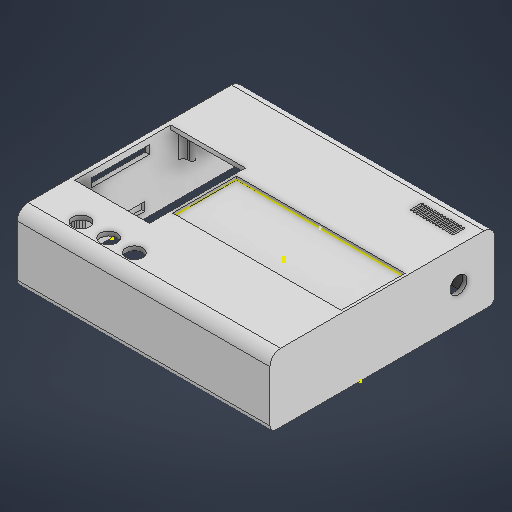
# Autodesk Inventor part: casereceptora
Saved by Autodesk Inventor 2026.1 (Build 301233020, 233B)
## iProperties
Created: 2025-11-04
Part Number: casereceptora
Material: Genérico
Document SubType Name: Modeling
Designer: luska
Density: 1 g/cm^3
Appearance: Padrão
Author: luska
## iProperties of the stored document casereceptora_3DPrint.ipt
Created: 2025-11-11
Part Number: casereceptora_3DPrint
Material: Genérico
Document SubType Name: Modeling
Designer: luska
Density: 1 g/cm^3
Appearance: Padrão
Author: luska
Autodesk Inventor part; units mm, degrees
ref_plane "YZ Plane" through (0, 0, 0) normal (1, 0, 0) x (0, 1, 0)
ref_plane "XZ Plane" through (0, 0, 0) normal (0, 1, 0) x (-1, 0, 0)
ref_plane "XY Plane" through (0, 0, 0) normal (0, 0, 1) x (1, 0, 0)
sketch "Esboço1" plane through (0, 0, 0) normal (0, 1, 0) x (-1, 0, 0)
  line L0 (82.792, 42.4072) -> (-35.708, 42.4072)
  line L1 (-35.708, 42.4072) -> (-35.708, -63.0628)
  line L2 (-35.708, -63.0628) -> (82.792, -63.0628)
  line L3 (82.792, -63.0628) -> (82.792, 42.4072)
  point P0 (0, 0)
  constraints: 8 end point, 2 parallel, 1 horizontal, 1 perpendicular
extrude "Extrusão1" add sketch "Esboço1" along normal blind 32
sketch "Esboço2" plane through (0, 0, 0) normal (0, -1, 0) x (1, 0, 0)
  line L0 (-80.792, 39.4072) -> (33.708, 39.4072)
  line L1 (33.708, 39.4072) -> (33.708, -60.0628)
  line L2 (33.708, -60.0628) -> (-80.792, -60.0628)
  line L3 (-80.792, -60.0628) -> (-80.792, 39.4072)
  line L4 (-82.792, -63.0628) -> (-82.792, 42.4072) projected
  line L5 (35.708, 42.4072) -> (35.708, -63.0628) projected
  line L6 (-82.792, 42.4072) -> (35.708, 42.4072) projected
  line L7 (35.708, -63.0628) -> (-82.792, -63.0628) projected
  point P0 (0, 0)
  constraints: 8 end point, 2 parallel, 1 horizontal, 1 perpendicular
extrude "Extrusão2" cut sketch "Esboço2" against normal blind 30 contours L0 L1 L2 L3
sketch "Esboço3" plane through (-82.792, 0, -63.0628) normal (-1, 0, 0) x (0, 0, 1)
  line L0 (24.47, 25) -> (14.47, 25)
  line L1 (14.47, 25) -> (14.47, 20)
  line L2 (14.47, 20) -> (24.47, 20)
  line L3 (24.47, 20) -> (24.47, 25)
  line L4 (0, 32) -> (105.47, 32) projected
  line L5 (0, 0) -> (0, 32) projected
  line L6 (45.47, 25) -> (72.47, 25)
  line L7 (72.47, 25) -> (72.47, 29)
  line L8 (72.47, 29) -> (45.47, 29)
  line L9 (45.47, 29) -> (45.47, 25)
  line L10 (105.47, 0) -> (105.47, 32) projected
  point P0 (63.0628, 0)
  point P1 (19.47, 25)
  point P2 (14.47, 22.5)
  point P3 (52.735, 32)
  point P4 (72.47, 27)
  point P5 (45.47, 27)
  dimension "d12" = 10
  dimension "d13" = 5
  dimension "d16" = 27
  dimension "d17" = 4
  dimension "d18" = 3
  dimension "d19" = 33
  dimension "d269" = 21
  dimension "d273" = 7
  constraints: 16 end point, 5 midpoint, 4 parallel, 2 horizontal, 2 perpendicular
  measures "d12" distance of L2.end L1.end
  measures "d13" distance of L1.end L0.end
  measures "d16" distance of L8.end L7.end
  measures "d17" distance of L7.end L6.end
  measures "d18" distance from line of point (52.735, 32) L8
  measures "d19" distance from line of L10 point (72.47, 27)
  measures "d269" distance from line of point (45.47, 27) L3
  measures "d273" distance between parallel lines of L4 L0
extrude "Extrusão3" cut sketch "Esboço3" against normal blind 2
sketch "Esboço4" plane through (0, 30, 0) normal (0, -1, 0) x (1, 0, 0)
  point P0 (0, 0)
sketch "Esboço5" plane through (0, 30, 0) normal (0, -1, 0) x (1, 0, 0)
  line L0 (-45.792, -27.5928) -> (-80.792, -27.5928)
  line L1 (-80.792, -27.5928) -> (-80.792, 17.4072)
  line L2 (-80.792, 17.4072) -> (-45.792, 17.4072)
  line L3 (-45.792, 17.4072) -> (-45.792, -27.5928)
  line L4 (-82.792, -63.0628) -> (-82.792, 42.4072) projected
  line L5 (-82.792, 42.4072) -> (35.708, 42.4072) projected
  line L6 (-80.792, 39.4072) -> (33.708, 39.4072) projected
  point P0 (0, 0)
  point P1 (-63.292, 17.4072)
  dimension "d22" = 35
  dimension "d23" = 45
  dimension "d24" = 2
  dimension "d268" = 22
  constraints: 8 end point, 2 parallel, 1 horizontal, 1 midpoint, 1 perpendicular
  measures "d22" distance of L1.end L2.end
  measures "d23" distance from line of point (-63.292, 17.407) L0
  measures "d24" distance between parallel lines of L4 L1
  measures "d268" distance between parallel lines of L6 L2
extrude "Extrusão4" cut sketch "Esboço5" against normal blind 2
sketch "Esboço6" plane through (0, 30, 0) normal (0, -1, 0) x (1, 0, 0)
  circle A0 centre (-78.392, 36.4072) radius 1.5
  line L0 (-80.792, -60.0628) -> (-80.792, 39.4072) projected
  line L1 (-80.792, 39.4072) -> (33.708, 39.4072) projected
  circle A1 centre (24.108, 35.4072) radius 1.25
  circle A2 centre (25.208, -54.0928) radius 1.25
  circle A3 centre (-77.792, -34.5928) radius 1.25
  line L2 (33.708, -60.0628) -> (-80.792, -60.0628) projected
  point P0 (0, 0)
  dimension "d28" = 3
  dimension "d29" = 2.4
  dimension "d30" = 3
  dimension "d32" = 2.5
  dimension "d33" = 2.5
  dimension "d34" = 2.5
  dimension "d35" = 4
  dimension "d39" = 3
  dimension "d249" = 102.5
  dimension "d250" = 71
  dimension "d251" = 89.5
  dimension "d261" = 106
  constraints: 4 centre point
  measures "d28" diameter of A0
  measures "d29" distance from line of L0 A0.centre
  measures "d30" distance from line of A0.centre L1
  measures "d32" diameter of A1
  measures "d33" diameter of A2
  measures "d34" diameter of A3
  measures "d35" distance from line of L1 A1.centre
  measures "d39" distance from line of L0 A3.centre
  measures "d249" horizontal distance of A0.centre A1.centre
  measures "d250" vertical distance of A3.centre A0.centre
  measures "d251" vertical distance of A1.centre A2.centre
  measures "d261" distance from line of L0 A2.centre
extrude "Extrusão5" add sketch "Esboço6" along normal blind 14
fillet "Arredondamento1" radius 5 2 edges at (-23.542, 32, 42.4072) (-23.542, 32, -63.0628)
fillet "Arredondamento2" radius 3 2 edges at (-23.542, 0, -63.0628) (-23.542, 0, 42.4072)
sketch "Esboço8" plane through (0, 32, 0) normal (0, 1, 0) x (1, 0, 0)
  line L0 (-65.977, -29.8737) -> (-62.9265, -29.8737) construction
  line L1 (-62.9265, -29.8737) -> (-62.9265, -32.2177) construction
  line L2 (-62.9265, -32.2177) -> (-65.977, -32.2177) construction
  line L3 (-65.977, -32.2177) -> (-65.977, -29.8737) construction
  line L4 (-52.6086, -29.9418) -> (-49.5581, -29.9418) construction
  line L5 (-49.5581, -29.9418) -> (-49.5581, -32.2859) construction
  line L6 (-49.5581, -32.2859) -> (-52.6086, -32.2859) construction
  line L7 (-52.6086, -32.2859) -> (-52.6086, -29.9418) construction
  arc A0 (-37.9057, -29.1205) -> (-36.0322, -29.1205) centre (-36.9689, -31.1663) ccw
  line L8 (-49.9706, -31.2361) -> (-52.169, -32.2859)
  line L9 (-52.169, -32.2859) -> (-52.169, -31.9228)
  line L10 (-52.169, -31.9228) -> (-50.4646, -31.1126)
  line L11 (-50.4646, -31.1126) -> (-52.169, -30.3049)
  line L12 (-52.169, -30.3049) -> (-52.169, -29.9418)
  line L13 (-52.169, -29.9418) -> (-49.9706, -30.9916)
  line L14 (-49.9706, -30.9916) -> (-49.9706, -31.2361)
  line L15 (-63.3662, -32.2177) -> (-65.5645, -31.1679)
  line L16 (-65.5645, -31.1679) -> (-65.5645, -30.9234)
  line L17 (-65.5645, -30.9234) -> (-63.3662, -29.8737)
  line L18 (-63.3662, -29.8737) -> (-63.3662, -30.2368)
  line L19 (-63.3662, -30.2368) -> (-65.0705, -31.0444)
  line L20 (-65.0705, -31.0444) -> (-63.3662, -31.8546)
  line L21 (-63.3662, -31.8546) -> (-63.3662, -32.2177)
  point P0 (0, 0)
  point P1 (-36.9689, -33.4163)
  constraints: 3 point on circle, 1 centre point, 4 other
extrude "Extrusão7" add sketch "Esboço8" against normal blind 1
sketch "Esboço11" plane through (0, 32, 0) normal (0, 1, 0) x (1, 0, 0)
  point P0 (0, 0)
sketch "Esboço12" plane through (0, 32, 0) normal (0, 1, 0) x (1, 0, 0)
  line L0 (-44.5183, -7.7581) -> (34.4817, -7.7581)
  line L1 (34.4817, -7.7581) -> (34.4817, 22.2419)
  line L2 (34.4817, 22.2419) -> (-44.5183, 22.2419)
  line L3 (-44.5183, 22.2419) -> (-44.5183, -7.7581)
  point P0 (0, 0)
  dimension "d236" = 79
  dimension "d237" = 30
  constraints: 8 end point, 2 parallel, 1 horizontal, 1 perpendicular
  measures "d236" distance between parallel lines of L1 L3
  measures "d237" distance between parallel lines of L0 L2
extrude "Extrusão9" cut sketch "Esboço12" against normal blind 1.5
sketch "Esboço14" plane through (0, 32, 0) normal (0, 1, 0) x (1, 0, 0)
  line L0 (29.7829, 54.3851) -> (29.7829, 49.3588) construction
  line L1 (29.3347, 54.3851) -> (29.3347, 49.3588)
  line L2 (30.231, 49.3588) -> (30.231, 54.3851)
  arc A0 (30.231, 54.3851) -> (29.3347, 54.3851) centre (29.7829, 54.3851) ccw
  arc A1 (29.3347, 49.3588) -> (30.231, 49.3588) centre (29.7829, 49.3588) ccw
  line L3 (28.2829, 54.3851) -> (28.2829, 49.3588) construction
  line L4 (27.8347, 54.3851) -> (27.8347, 49.3588)
  line L5 (28.731, 49.3588) -> (28.731, 54.3851)
  arc A2 (28.731, 54.3851) -> (27.8347, 54.3851) centre (28.2829, 54.3851) ccw
  arc A3 (27.8347, 49.3588) -> (28.731, 49.3588) centre (28.2829, 49.3588) ccw
  line L6 (23.7829, 54.3851) -> (23.7829, 49.3588) construction
  line L7 (23.3347, 54.3851) -> (23.3347, 49.3588)
  line L8 (24.231, 49.3588) -> (24.231, 54.3851)
  arc A4 (24.231, 54.3851) -> (23.3347, 54.3851) centre (23.7829, 54.3851) ccw
  arc A5 (23.3347, 49.3588) -> (24.231, 49.3588) centre (23.7829, 49.3588) ccw
  line L9 (22.2829, 54.3851) -> (22.2829, 49.3588) construction
  line L10 (21.8347, 54.3851) -> (21.8347, 49.3588)
  line L11 (22.731, 49.3588) -> (22.731, 54.3851)
  arc A6 (22.731, 54.3851) -> (21.8347, 54.3851) centre (22.2829, 54.3851) ccw
  arc A7 (21.8347, 49.3588) -> (22.731, 49.3588) centre (22.2829, 49.3588) ccw
  line L12 (17.7829, 54.3851) -> (17.7829, 49.3588) construction
  line L13 (17.3347, 54.3851) -> (17.3347, 49.3588)
  line L14 (18.231, 49.3588) -> (18.231, 54.3851)
  arc A8 (18.231, 54.3851) -> (17.3347, 54.3851) centre (17.7829, 54.3851) ccw
  arc A9 (17.3347, 49.3588) -> (18.231, 49.3588) centre (17.7829, 49.3588) ccw
  line L15 (16.2829, 54.3851) -> (16.2829, 49.3588) construction
  line L16 (15.8347, 54.3851) -> (15.8347, 49.3588)
  line L17 (16.731, 49.3588) -> (16.731, 54.3851)
  arc A10 (16.731, 54.3851) -> (15.8347, 54.3851) centre (16.2829, 54.3851) ccw
  arc A11 (15.8347, 49.3588) -> (16.731, 49.3588) centre (16.2829, 49.3588) ccw
  line L18 (14.7829, 54.3851) -> (14.7829, 49.3588) construction
  line L19 (14.3347, 54.3851) -> (14.3347, 49.3588)
  line L20 (15.231, 49.3588) -> (15.231, 54.3851)
  arc A12 (15.231, 54.3851) -> (14.3347, 54.3851) centre (14.7829, 54.3851) ccw
  arc A13 (14.3347, 49.3588) -> (15.231, 49.3588) centre (14.7829, 49.3588) ccw
  line L21 (13.2829, 54.3851) -> (13.2829, 49.3588) construction
  line L22 (12.8347, 54.3851) -> (12.8347, 49.3588)
  line L23 (13.731, 49.3588) -> (13.731, 54.3851)
  arc A14 (13.731, 54.3851) -> (12.8347, 54.3851) centre (13.2829, 54.3851) ccw
  arc A15 (12.8347, 49.3588) -> (13.731, 49.3588) centre (13.2829, 49.3588) ccw
  line L24 (20.7829, 54.3851) -> (20.7829, 49.3588) construction
  line L25 (20.3347, 54.3851) -> (20.3347, 49.3588)
  line L26 (21.231, 49.3588) -> (21.231, 54.3851)
  arc A16 (21.231, 54.3851) -> (20.3347, 54.3851) centre (20.7829, 54.3851) ccw
  arc A17 (20.3347, 49.3588) -> (21.231, 49.3588) centre (20.7829, 49.3588) ccw
  line L27 (19.2829, 54.3851) -> (19.2829, 49.3588) construction
  line L28 (18.8347, 54.3851) -> (18.8347, 49.3588)
  line L29 (19.731, 49.3588) -> (19.731, 54.3851)
  arc A18 (19.731, 54.3851) -> (18.8347, 54.3851) centre (19.2829, 54.3851) ccw
  arc A19 (18.8347, 49.3588) -> (19.731, 49.3588) centre (19.2829, 49.3588) ccw
  line L30 (26.7829, 54.3851) -> (26.7829, 49.3588) construction
  line L31 (26.3347, 54.3851) -> (26.3347, 49.3588)
  line L32 (27.231, 49.3588) -> (27.231, 54.3851)
  arc A20 (27.231, 54.3851) -> (26.3347, 54.3851) centre (26.7829, 54.3851) ccw
  arc A21 (26.3347, 49.3588) -> (27.231, 49.3588) centre (26.7829, 49.3588) ccw
  line L33 (25.2829, 54.3851) -> (25.2829, 49.3588) construction
  line L34 (24.8347, 54.3851) -> (24.8347, 49.3588)
  line L35 (25.731, 49.3588) -> (25.731, 54.3851)
  arc A22 (25.731, 54.3851) -> (24.8347, 54.3851) centre (25.2829, 54.3851) ccw
  arc A23 (24.8347, 49.3588) -> (25.731, 49.3588) centre (25.2829, 49.3588) ccw
  line L36 (11.7829, 54.3851) -> (11.7829, 49.3588) construction
  line L37 (11.3347, 54.3851) -> (11.3347, 49.3588)
  line L38 (12.231, 49.3588) -> (12.231, 54.3851)
  arc A24 (12.231, 54.3851) -> (11.3347, 54.3851) centre (11.7829, 54.3851) ccw
  arc A25 (11.3347, 49.3588) -> (12.231, 49.3588) centre (11.7829, 49.3588) ccw
  line L39 (10.2829, 54.3851) -> (10.2829, 49.3588) construction
  line L40 (9.8347, 54.3851) -> (9.8347, 49.3588)
  line L41 (10.731, 49.3588) -> (10.731, 54.3851)
  arc A26 (10.731, 54.3851) -> (9.8347, 54.3851) centre (10.2829, 54.3851) ccw
  arc A27 (9.8347, 49.3588) -> (10.731, 49.3588) centre (10.2829, 49.3588) ccw
  point P0 (0, 0)
  point P1 (29.7829, 51.872)
  point P2 (28.2829, 51.872)
  point P3 (23.7829, 51.872)
  point P4 (22.2829, 51.872)
  point P5 (17.7829, 51.872)
  point P6 (16.2829, 51.872)
  point P7 (14.7829, 51.872)
  point P8 (13.2829, 51.872)
  point P9 (20.7829, 51.872)
  point P10 (19.2829, 51.872)
  point P11 (26.7829, 51.872)
  point P12 (25.2829, 51.872)
  point P13 (11.7829, 51.872)
  point P14 (10.2829, 51.872)
  constraints: 112 end point, 56 point on circle, 56 tangent, 28 centre point, 14 midpoint, 14 parallel, 14 vertical
extrude "Extrusão11" cut sketch "Esboço14" against normal blind 2
sketch "Esboço15" plane through (-82.792, 32, -58.0628) normal (-1, 0, 0) x (0, 0, 1)
  line L0 (71.2913, -27) -> (71.2913, -7) construction
  line L1 (72.0413, -26.25) -> (72.0413, -7.75)
  line L2 (70.5413, -7.75) -> (70.5413, -26.25)
  arc A0 (70.5413, -26.25) -> (72.0413, -26.25) centre (71.2913, -26.25) ccw
  arc A1 (72.0413, -7.75) -> (70.5413, -7.75) centre (71.2913, -7.75) ccw
  line L3 (0, 0) -> (95.47, 0) projected
  line L4 (73.8106, -27) -> (73.8106, -7) construction
  line L5 (74.5606, -26.25) -> (74.5606, -7.75)
  line L6 (73.0606, -7.75) -> (73.0606, -26.25)
  arc A2 (73.0606, -26.25) -> (74.5606, -26.25) centre (73.8106, -26.25) ccw
  arc A3 (74.5606, -7.75) -> (73.0606, -7.75) centre (73.8106, -7.75) ccw
  line L7 (76.2114, -27) -> (76.2114, -7) construction
  line L8 (76.9614, -26.25) -> (76.9614, -7.75)
  line L9 (75.4614, -7.75) -> (75.4614, -26.25)
  arc A4 (75.4614, -26.25) -> (76.9614, -26.25) centre (76.2114, -26.25) ccw
  arc A5 (76.9614, -7.75) -> (75.4614, -7.75) centre (76.2114, -7.75) ccw
  line L10 (78.5611, -27) -> (78.5611, -7) construction
  line L11 (79.3111, -26.25) -> (79.3111, -7.75)
  line L12 (77.8111, -7.75) -> (77.8111, -26.25)
  arc A6 (77.8111, -26.25) -> (79.3111, -26.25) centre (78.5611, -26.25) ccw
  arc A7 (79.3111, -7.75) -> (77.8111, -7.75) centre (78.5611, -7.75) ccw
  line L13 (80.9109, -27) -> (80.9109, -7) construction
  line L14 (81.6609, -26.25) -> (81.6609, -7.75)
  line L15 (80.1609, -7.75) -> (80.1609, -26.25)
  arc A8 (80.1609, -26.25) -> (81.6609, -26.25) centre (80.9109, -26.25) ccw
  arc A9 (81.6609, -7.75) -> (80.1609, -7.75) centre (80.9109, -7.75) ccw
  line L16 (83.4649, -27) -> (83.4649, -7) construction
  line L17 (84.2149, -26.25) -> (84.2149, -7.75)
  line L18 (82.7149, -7.75) -> (82.7149, -26.25)
  arc A10 (82.7149, -26.25) -> (84.2149, -26.25) centre (83.4649, -26.25) ccw
  arc A11 (84.2149, -7.75) -> (82.7149, -7.75) centre (83.4649, -7.75) ccw
  line L19 (86.07, -27) -> (86.07, -7) construction
  line L20 (86.82, -26.25) -> (86.82, -7.75)
  line L21 (85.32, -7.75) -> (85.32, -26.25)
  arc A12 (85.32, -26.25) -> (86.82, -26.25) centre (86.07, -26.25) ccw
  arc A13 (86.82, -7.75) -> (85.32, -7.75) centre (86.07, -7.75) ccw
  line L22 (68.9579, -27) -> (68.9579, -7) construction
  line L23 (88.4709, -27) -> (88.4709, -7) construction
  line L24 (89.2209, -26.25) -> (89.2209, -7.75)
  line L25 (87.7209, -7.75) -> (87.7209, -26.25)
  arc A14 (87.7209, -26.25) -> (89.2209, -26.25) centre (88.4709, -26.25) ccw
  arc A15 (89.2209, -7.75) -> (87.7209, -7.75) centre (88.4709, -7.75) ccw
  point P0 (58.0628, -32)
  point P1 (71.2913, -17)
  point P2 (71.2913, -7)
  point P3 (73.8106, -17)
  point P4 (73.8106, -7)
  point P5 (76.2114, -17)
  point P6 (76.2114, -7)
  point P7 (78.5611, -17)
  point P8 (78.5611, -7)
  point P9 (80.9109, -17)
  point P10 (80.9109, -7)
  point P11 (83.4649, -17)
  point P12 (83.4649, -7)
  point P13 (86.07, -17)
  point P14 (86.07, -7)
  point P15 (88.4709, -17)
  point P16 (88.4709, -7)
  constraints: 68 end point, 56 point on circle, 32 tangent, 16 centre point, 16 point on line, 9 vertical, 8 midpoint, 8 parallel
extrude "Extrusão12" cut sketch "Esboço15" against normal blind 2
sketch "Esboço17" plane through (0, 30.5, 0) normal (0, 1, 0) x (1, 0, 0)
  point P0 (0, 0)
sketch "Esboço18" plane through (0, 30, 0) normal (0, -1, 0) x (1, 0, 0)
  point P0 (0, 0)
sketch "Esboço21" plane through (33.708, 30, -60.0628) normal (-1, 0, 0) x (0, 0, 1)
  point P0 (60.0628, -30)
sketch "Esboço22" plane through (35.708, 32, 37.4072) normal (1, 0, 0) x (0, 0, -1)
  point P0 (37.4072, -32)
sketch "Esboço27" plane through (0, 30.5, 0) normal (0, 1, 0) x (1, 0, 0)
  line L0 (-44.5183, -7.7581) -> (-44.5183, 22.2419) projected
  line L1 (-44.5183, 22.2419) -> (34.4817, 22.2419) projected
  line L2 (34.4817, -7.7581) -> (-44.5183, -7.7581) projected
  point P0 (0, 0)
  point P1 (-5.0183, 22.2419)
  point P2 (-5.0183, -7.7581)
  constraints: 2 midpoint
sketch "Esboço29" plane through (35.708, 27, -63.0628) normal (0, 0, -1) x (-1, 0, 0)
  point P0 (35.708, -27)
sketch "Esboço30" plane through (-82.792, 32, -58.0628) normal (-1, 0, 0) x (0, 0, 1)
  point P0 (58.0628, -32)
sketch "Esboço31" plane through (0, 30, 0) normal (0, -1, 0) x (1, 0, 0)
  point P0 (0, 0)
sketch "Esboço32" plane through (-80.792, 32, 17.4072) normal (1, 0, 0) x (0, 0, -1)
  point P0 (17.4072, -32)
sketch "Esboço33" plane through (0, 0, 0) normal (0, -1, 0) x (1, 0, 0)
  point P0 (0, 0)
sketch "Esboço37" plane through (25.208, 16, -54.0928) normal (0, -1, 0) x (1, 0, 0)
  circle A0 centre (0, 0) radius 0.75
  point P0 (-25.208, 54.0928)
  dimension "d189" = 1.5
  constraints: 1 centre point
  measures "d189" diameter of A0
extrude "Extrusão22" cut sketch "Esboço37" against normal blind 5
sketch "Esboço38" plane through (-77.792, 16, -34.5928) normal (0, -1, 0) x (1, 0, 0)
  circle A0 centre (0, 0) radius 0.75
  point P0 (77.792, 34.5928)
  dimension "d192" = 1.5
  constraints: 1 centre point
  measures "d192" diameter of A0
extrude "Extrusão23" cut sketch "Esboço38" against normal blind 5
sketch "Esboço39" plane through (-78.392, 16, 36.4072) normal (0, -1, 0) x (1, 0, 0)
  circle A0 centre (0, 0) radius 0.75
  point P0 (78.392, -36.4072)
  dimension "d195" = 1.5
  constraints: 1 centre point
  measures "d195" diameter of A0
extrude "Extrusão24" cut sketch "Esboço39" against normal blind 5
sketch "Esboço40" plane through (24.108, 16, 35.4072) normal (0, -1, 0) x (1, 0, 0)
  circle A0 centre (0, 0) radius 0.75
  point P0 (-24.108, -35.4072)
  dimension "d198" = 1.5
  constraints: 1 centre point
  measures "d198" diameter of A0
extrude "Extrusão25" cut sketch "Esboço40" against normal blind 5
sketch "Esboço42" plane through (-80.792, 32, 17.4072) normal (1, 0, 0) x (0, 0, -1)
  point P0 (17.4072, -32)
sketch "Esboço43" plane through (-80.792, 32, 17.4072) normal (1, 0, 0) x (0, 0, -1)
  line L0 (32.735, -25) -> (22.735, -25)
  line L1 (22.735, -25) -> (22.735, -29)
  line L2 (22.735, -29) -> (32.735, -29)
  line L3 (32.735, -29) -> (32.735, -25)
  line L4 (77.47, -32) -> (-22, -32) projected
  line L5 (-22, -32) -> (-22, -2) projected
  point P0 (17.4072, -32)
  point P1 (22.735, -27)
  dimension "d206" = 10
  dimension "d207" = 4
  dimension "d208" = 3
  dimension "d209" = 44.735
  constraints: 8 end point, 2 parallel, 1 horizontal, 1 midpoint, 1 perpendicular
  measures "d206" distance of L2.end L1.end
  measures "d207" distance between parallel lines of L2 L0
  measures "d208" distance between parallel lines of L4 L2
  measures "d209" distance from line of point (22.735, -27) L5
extrude "Extrusão27" cut sketch "Esboço43" against normal blind 1.5
sketch "Esboço44" plane through (33.708, 30, -60.0628) normal (-1, 0, 0) x (0, 0, 1)
  line L0 (44.735, -28) -> (54.735, -28)
  line L1 (54.735, -28) -> (54.735, 0)
  line L2 (54.735, 0) -> (44.735, 0)
  line L3 (44.735, 0) -> (44.735, -28)
  line L4 (0, -30) -> (0, 0) projected
  line L5 (99.47, -30) -> (0, -30) projected
  point P0 (60.0628, -30)
  point P1 (44.735, -14)
  dimension "d212" = 10
  dimension "d213" = 28
  dimension "d214" = 44.735
  dimension "d230" = 2
  constraints: 8 end point, 2 parallel, 1 horizontal, 1 midpoint, 1 perpendicular
  measures "d212" distance of L2.end L1.end
  measures "d213" distance of L1.end L0.end
  measures "d214" distance from line of L4 point (44.735, -14)
  measures "d230" distance between parallel lines of L5 L0
extrude "Extrusão28" add sketch "Esboço44" along normal blind 4
sketch "Esboço45" plane through (33.708, 2, -15.3278) normal (0, -1, 0) x (1, 0, 0)
  circle A0 centre (-2, 5) radius 0.75
  line L0 (0, 0) -> (-4, 0) projected
  line L1 (-4, 0) -> (-4, 10) projected
  point P0 (-33.708, 15.3278)
  point P1 (-4, 5)
  dimension "d217" = 1.5
  dimension "d218" = 5
  dimension "d219" = 2
  constraints: 1 centre point, 1 midpoint
  measures "d217" diameter of A0
  measures "d218" distance from line of L0 A0.centre
  measures "d219" distance of point (-4, 5) A0.centre
extrude "Extrusão29" cut sketch "Esboço45" against normal blind 10
sketch "Esboço47" plane through (0, 30, 0) normal (0, -1, 0) x (1, 0, 0)
  circle A0 centre (25.208, -54.0928) radius 1.25 projected
  line L0 (23.958, -54.0928) -> (23.958, -56.5337)
  line L1 (26.458, -54.0928) -> (26.458, -56.5337)
  line L2 (26.458, -56.5337) -> (23.958, -56.5337)
  point P0 (0, 0)
  constraints: 6 end point, 2 point on circle, 2 tangent, 2 vertical, 1 perpendicular
extrude "Extrusão31" add sketch "Esboço47" along normal blind 14 contours L1 L2 L0 A0
sketch "Esboço48" plane through (0, 30, 0) normal (0, -1, 0) x (1, 0, 0)
  circle A0 centre (24.108, 35.4072) radius 1.25 projected
  line L0 (25.358, 35.4072) -> (25.358, 39.4072)
  line L1 (-80.792, 39.4072) -> (33.708, 39.4072) projected
  circle A1 centre (-78.392, 36.4072) radius 1.5 projected
  line L2 (-76.892, 36.4072) -> (-76.892, 39.4072)
  line L3 (-79.892, 36.4072) -> (-79.892, 39.4072)
  circle A2 centre (-77.792, -34.5928) radius 1.25 projected
  line L4 (-77.792, -35.8428) -> (-81.092, -35.8428)
  line L5 (-77.792, -33.3428) -> (-80.792, -33.3428)
  line L6 (-80.792, -60.0628) -> (-80.792, -27.5928) projected
  line L7 (22.858, 35.4072) -> (22.858, 39.4072)
  point P0 (0, 0)
  point P1 (-80.792, -27.5928)
  point P2 (-80.792, -35.8428)
  constraints: 12 end point, 6 point on circle, 4 point on line, 3 perpendicular, 3 tangent, 2 horizontal, 1 vertical, 2 other
extrude "Extrusão32" add sketch "Esboço48" along normal blind 14 contours A0 L7 L1 L0 | L1 L2 A1 L3 | A2 L4 L6 L5
fillet "Arredondamento4" radius 2 2 edges at (29.708, 16, -5.3278) (29.708, 16, -15.3278)
sketch "Esboço49" plane through (0, 30, 0) normal (0, -1, 0) x (1, 0, 0)
  circle A0 centre (-62.392, 32.9072) radius 4
  circle A1 centre (-37.392, 32.9072) radius 4
  circle A2 centre (-49.392, 32.9072) radius 4
  circle A3 centre (-78.392, 36.4072) radius 0.75 projected
  line L0 (-80.792, 39.4072) -> (33.708, 39.4072) projected
  point P0 (0, 0)
  dimension "d238" = 8
  dimension "d239" = 8
  dimension "d240" = 8
  dimension "d241" = 16
  dimension "d242" = 6.5
  dimension "d243" = 13
  dimension "d244" = 12
  dimension "d245" = 6.5
  dimension "d246" = 6.5
  constraints: 3 centre point
  measures "d238" diameter of A0
  measures "d239" diameter of A1
  measures "d240" diameter of A2
  measures "d241" horizontal distance of A3.centre A0.centre
  measures "d242" distance from line of L0 A0.centre
  measures "d243" distance of A0.centre A2.centre
  measures "d244" distance of A1.centre A2.centre
  measures "d245" distance from line of L0 A2.centre
  measures "d246" distance from line of L0 A1.centre
extrude "Extrusão33" cut sketch "Esboço49" against normal blind 2 contours A0 | A1 | A2
sketch "Esboço50" plane through (35.708, 32, 37.4072) normal (1, 0, 0) x (0, 0, -1)
  circle A0 centre (83.47, -16) radius 4
  line L0 (100.47, -29) -> (100.47, -5) projected
  line L1 (0, 0) -> (95.47, 0) projected
  point P0 (37.4072, -32)
  dimension "d253" = 8
  dimension "d254" = 17
  dimension "d255" = 16
  constraints: 1 centre point
  measures "d253" diameter of A0
  measures "d254" distance from line of L0 A0.centre
  measures "d255" distance from line of L1 A0.centre
extrude "Extrusão34" cut sketch "Esboço50" against normal blind 2
sketch "Esboço51" plane through (33.708, 0, -60.0628) normal (-1, 0, 0) x (0, 0, 1)
  line L0 (22.325, 10.0916) -> (0, 10.0916)
  line L1 (0, 10.0916) -> (0, 21.9895)
  line L2 (0, 21.9895) -> (22.325, 21.9895)
  line L3 (22.325, 21.9895) -> (22.325, 10.0916)
  line L4 (0, 0) -> (0, 30) projected
  point P0 (60.0628, 0)
  dimension "d258" = 0
  constraints: 8 end point, 2 parallel, 1 horizontal, 1 perpendicular
  measures "d258" distance between parallel lines of L4 L1
extrude "Extrusão35" add sketch "Esboço51" along normal blind 6
sketch "Esboço52" plane through (33.708, 10.0916, -60.0628) normal (0, -1, 0) x (1, 0, 0)
  line L0 (0, 44.735) -> (0, 0) projected
  line L1 (-5.5, 17.925) -> (0, 17.925)
  line L2 (0, 17.925) -> (0, 9.925)
  line L3 (0, 9.925) -> (-5.5, 9.925)
  line L4 (-5.5, 9.925) -> (-5.5, 17.925)
  line L5 (-6, 0) -> (-6, 22.325) projected
  line L6 (0, 22.325) -> (-6, 22.325) projected
  point P0 (-33.708, 60.0628)
  point P1 (0, 17.925)
  dimension "d262" = 0.5
  dimension "d263" = 8
  dimension "d264" = 4.4
  constraints: 8 end point, 2 parallel, 1 horizontal, 1 perpendicular, 1 point on line
  measures "d262" distance between parallel lines of L5 L4
  measures "d263" distance between parallel lines of L1 L3
  measures "d264" distance between parallel lines of L6 L1
extrude "Extrusão36" cut sketch "Esboço52" against normal blind 17
sketch "Esboço53" plane through (0, 30, 0) normal (0, -1, 0) x (1, 0, 0)
  line L0 (26.458, -54.6938) -> (26.458, -56.5337) projected
  line L1 (33.708, -60.0628) -> (-80.792, -60.0628) projected
  line L2 (26.458, -56.5337) -> (23.979, -56.5337)
  line L3 (23.979, -56.5337) -> (23.979, -60.0628)
  line L4 (23.979, -60.0628) -> (26.458, -60.0628)
  line L5 (26.458, -60.0628) -> (26.458, -56.5337)
  point P0 (0, 0)
  constraints: 8 end point, 2 parallel, 1 horizontal, 1 perpendicular, 1 point on line
extrude "Extrusão37" add sketch "Esboço53" along normal blind 14
fillet "Arredondamento6" radius 2 10 edges at (33.708, 16.0406, -37.7378) (27.708, 16.0406, -37.7378) (23.979, 23, -60.0628) (27.708, 16.0406, -60.0628) (26.458, 23, -60.0628) (22.858, 23, 39.4072) (25.358, 23, 39.4072) (-76.892, 23, 39.4072) (-80.792, 23, -35.8428) (-80.792, 23, -33.3428)
